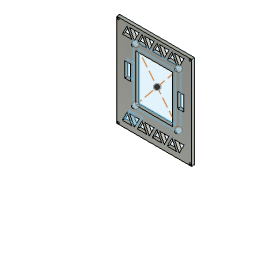
back_board (Autodesk Fusion 360 design; units mm, degrees)
Autodesk Fusion 360 part; units mm, degrees
ref_plane "WorkPlane1" through (0, 35, 0) normal (0, 1, 0) x (0, 0, 1)
sketch "Sketch1" plane through (0, 35, 0) normal (0, 1, 0) x (1, 0, 0)
  line L0 (50, -124) -> (-50, -124)
  line L1 (-50, -124) -> (-50, 0)
  line L2 (-50, 0) -> (50, 0)
  line L3 (50, 0) -> (50, -124)
  constraint horizontal L0
  constraint vertical L1
  constraint horizontal L2
  constraint vertical L3
extrude "Extrude1" add sketch "Sketch1" along normal blind 4
sketch "Sketch2" plane through (0, 39, 0) normal (0, 1, 0) x (-1, 0, 0)
  line L0 (-50, 0) -> (50, 0)
  line L1 (50, 0) -> (50, 124)
  line L2 (50, 124) -> (-50, 124)
  line L3 (-50, 124) -> (-50, 0)
  circle A0 centre (48, 122) radius 1.2
  circle A1 centre (48, 2) radius 1.2
  circle A2 centre (-48, 2) radius 1.2
  circle A3 centre (-48, 122) radius 1.2
  dimension "d149" = 2.4
  dimension "d150" = 2
  dimension "d151" = 2
  dimension "d152" = 2.4
  dimension "d153" = 2
  dimension "d154" = 2
  dimension "d155" = 2.4
  dimension "d156" = 2
  dimension "d157" = 2
  dimension "d158" = 2.4
  dimension "d159" = 2
  dimension "d160" = 2
  measures "d149" diameter of A0
  measures "d150" distance of L2 A0.centre
  measures "d151" distance of L1 A0.centre
  measures "d152" diameter of A1
  measures "d153" distance of L1 A1.centre
  measures "d154" distance of L0 A1.centre
  measures "d155" diameter of A2
  measures "d156" distance of L0 A2.centre
  measures "d157" distance of L3 A2.centre
  measures "d158" diameter of A3
  measures "d159" distance of L3 A3.centre
  measures "d160" distance of L2 A3.centre
extrude "Extrude2" cut sketch "Sketch2" against normal blind 4 contours A0 | A1 | A2 | A3
sketch "Sketch3" plane through (0, 39, 0) normal (0, 1, 0) x (-1, 0, 0)
  circle A0 centre (48, 122) radius 1.2
  circle A1 centre (48, 2) radius 1.2
  circle A2 centre (-48, 122) radius 1.2
  circle A3 centre (-48, 2) radius 1.2
  line L0 (-50, 0) -> (50, 0)
  line L1 (50, 0) -> (50, 124)
  line L2 (50, 124) -> (-50, 124)
  line L3 (-50, 124) -> (-50, 0)
  line L4 (31.5, 26.5) -> (-31.5, 26.5)
  line L5 (-31.5, 26.5) -> (-31.5, 103.5)
  line L6 (-31.5, 103.5) -> (31.5, 103.5)
  line L7 (31.5, 103.5) -> (31.5, 26.5)
  line L8 (31.5, 26.5) -> (-31.5, 103.5) construction
  line L9 (-31.5, 26.5) -> (31.5, 103.5) construction
  line L10 (24.5, 33.5) -> (-24.5, 33.5)
  line L11 (-24.5, 33.5) -> (-24.5, 96.5)
  line L12 (-24.5, 96.5) -> (24.5, 96.5)
  line L13 (24.5, 96.5) -> (24.5, 33.5)
  circle A4 centre (28.8, 100.8) radius 1.55
  circle A5 centre (28.8, 29.2) radius 1.55
  circle A6 centre (-28.8, 29.2) radius 1.55
  circle A7 centre (-28.8, 100.8) radius 1.55
  line L14 (31.5, 77.6587) -> (39.5, 77.6587)
  line L15 (39.5, 77.6587) -> (39.5, 57.6587)
  line L16 (39.5, 57.6587) -> (31.5, 57.6587)
  line L17 (31.5, 57.6587) -> (31.5, 77.6587)
  point P0 (0, 65)
  dimension "d163" = 63
  dimension "d164" = 77
  dimension "d165" = 7
  dimension "d168" = 3.1
  dimension "d169" = 2.7
  dimension "d170" = 2.7
  dimension "d171" = 3.1
  dimension "d172" = 2.7
  dimension "d173" = 2.7
  dimension "d174" = 3.1
  dimension "d175" = 2.7
  dimension "d176" = 2.7
  dimension "d177" = 3.1
  dimension "d178" = 2.7
  dimension "d179" = 2.7
  dimension "d182" = 8
  dimension "d183" = 20
  constraint horizontal L4
  constraint perpendicular L4 L5
  constraint parallel L4 L6
  constraint parallel L5 L7
  constraint coincident L8 P0
  constraint coincident L9 P0
  constraint horizontal L14
  constraint vertical L15
  constraint horizontal L16
  constraint vertical L17
  constraint coincident L7 L14.start
  measures "d163" distance of L5.end L6.end
  measures "d164" distance of L4.end L5.end
  measures "d168" diameter of A4
  measures "d169" distance of L7 A4.centre
  measures "d170" distance of L6 A4.centre
  measures "d171" diameter of A5
  measures "d172" distance of L7 A5.centre
  measures "d173" distance of L4 A5.centre
  measures "d174" diameter of A6
  measures "d175" distance of L4 A6.centre
  measures "d176" distance of L5 A6.centre
  measures "d177" diameter of A7
  measures "d178" distance of L5 A7.centre
  measures "d179" distance of L6 A7.centre
  measures "d182" distance of L14.start L14.end
  measures "d183" distance of L14.start L16.end
extrude "Extrude3" cut sketch "Sketch3" against normal blind 4 contours L10 L11 L12 L13
extrude "Extrude4" cut sketch "Sketch3" against normal blind 4 contours A4 | A5 | A6 | A7
extrude "Extrude5" cut sketch "Sketch3" against normal blind 4 contours L7 L14 L15 L16 L17
mirror "Mirror1" about plane through (0, 0, 0) normal (1, 0, 0) of "Extrude5"
sketch "Sketch4" plane through (0, 39, 0) normal (0, 1, 0) x (-1, 0, 0)
  line L0 (-39.5, 57.6587) -> (-39.5, 77.6587)
  line L1 (-39.5, 77.6587) -> (-31.5, 77.6587)
  line L2 (-31.5, 77.6587) -> (-31.5, 57.6587)
  line L3 (-31.5, 57.6587) -> (-39.5, 57.6587)
  line L4 (39.5, 77.6587) -> (39.5, 57.6587)
  line L5 (39.5, 57.6587) -> (31.5, 57.6587)
  line L6 (31.5, 57.6587) -> (31.5, 77.6587)
  line L7 (31.5, 77.6587) -> (39.5, 77.6587)
  circle A0 centre (28.8, 100.8) radius 1.55
  circle A1 centre (28.8, 29.2) radius 1.55
  circle A2 centre (-28.8, 100.8) radius 1.55
  circle A3 centre (-28.8, 29.2) radius 1.55
  line L8 (-24.5, 33.5) -> (-24.5, 96.5)
  line L9 (-24.5, 96.5) -> (24.5, 96.5)
  line L10 (24.5, 96.5) -> (24.5, 33.5)
  line L11 (24.5, 33.5) -> (-24.5, 33.5)
  circle A4 centre (48, 122) radius 1.2
  circle A5 centre (48, 2) radius 1.2
  circle A6 centre (-48, 122) radius 1.2
  circle A7 centre (-48, 2) radius 1.2
  line L12 (-50, 0) -> (50, 0)
  line L13 (50, 0) -> (50, 124)
  line L14 (50, 124) -> (-50, 124)
  line L15 (-50, 124) -> (-50, 0)
  line L16 (42.5432, 7.1698) -> (30, 7.1698)
  line L17 (30, 7.1698) -> (36.2716, 19.5987)
  line L18 (36.2716, 19.5987) -> (42.5432, 7.1698)
  line L19 (20.1537, 19.5987) -> (32.6969, 19.5987)
  line L20 (32.6969, 19.5987) -> (26.4253, 7.1698)
  line L21 (26.4253, 7.1698) -> (20.1537, 19.5987)
  constraint parallel L12 L16
extrude "Extrude6" cut sketch "Sketch4" against normal blind 4 contours L16 L17 L18
extrude "Extrude7" cut sketch "Sketch4" against normal blind 4 contours L19 L20 L21
pattern_linear "R-Pattern1" count 4 spacing 20 along (1, 0, 0) count 2 spacing 100 along (0, 0, 1) of "Extrude6", "Extrude7"
